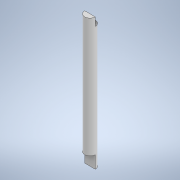
# Autodesk Inventor part: Twist_Rod
Saved by Autodesk Inventor 2022 (Build 260153000, 153)
## iProperties
Created: 2022-02-26
Part Number: Twist_Rod
Material: Generic
Document SubType Name: Modeling
Designer: Mlees
Density: 1 g/cm^3
Appearance: Default
Author: Mlees
Autodesk Inventor part; units mm, degrees
ref_plane "YZ Plane" through (0, 0, 0) normal (1, 0, 0) x (0, 1, 0)
ref_plane "XZ Plane" through (0, 0, 0) normal (0, 1, 0) x (-1, 0, 0)
ref_plane "XY Plane" through (0, 0, 0) normal (0, 0, 1) x (1, 0, 0)
sketch "Sketch1" plane through (0, 0, 0) normal (0, 1, 0) x (-1, 0, 0)
  circle A0 centre (0, 0) radius 2.625
  dimension "d0" = 5.25
  constraints: 1 centre point, 1 coincident
  measures "d0" diameter of A0
extrude "Extrusion1" add sketch "Sketch1" along normal blind 65
sketch "Sketch2" plane through (0, 65, 0) normal (0, 1, 0) x (1, 0, 0)
  circle A0 centre (0, 0) radius 2.625 projected
  line L0 (-2.625, 0) -> (2.625, 0)
  arc A1 (2.625, 0) -> (-2.625, 0) centre (0, 0) ccw
  constraints: 4 point on circle, 2 end point, 1 centre point, 1 concentric, 1 horizontal
extrude "Extrusion2" cut sketch "Sketch2" against normal blind 4 contours L0 A0 picked at (0.6549, 0.5802)
sketch "Sketch3" plane through (0, 0, 0) normal (0, -1, 0) x (1, 0, 0)
  arc A0 (2.625, 0) -> (-2.625, 0) centre (0, 0) ccw projected
  line L0 (2.625, 0) -> (-2.625, 0) projected
  line L1 (2.625, 0) -> (-2.625, 0)
  arc A1 (2.625, 0) -> (-2.625, 0) centre (0, 0) ccw
  constraints: 2 end point, 2 point on circle, 1 centre point, 1 collinear, 1 concentric
extrude "Extrusion3" cut sketch "Sketch3" against normal blind 6.2
body "Solid1"
